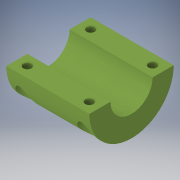
# Autodesk Inventor part: Slider Mount_B
Saved by Autodesk Inventor 2018 (Build 220112000, 112)
## iProperties
Created: 2018-01-05
Part Number: Slider Mount_B
Material: ABS Plastic
Document SubType Name: Modeling
Designer: njcfu
Density: 1.06 g/cm^3
Appearance: Olive Green
Author: njcfu
Autodesk Inventor part; units mm, degrees
sketch "Sketch2" plane through (0, 0, 0) normal (1, 0, 0) x (0, 1, 0)
  arc A0 (0, 12.7) -> (0, -12.7) centre (0, 0) ccw
  arc A1 (0, 25.4) -> (0, -25.4) centre (0, 0) ccw
  line L0 (0, -25.4) -> (0, -12.7)
  line L1 (0, 12.7) -> (0, 25.4)
  line L2 (0, 35.56) -> (0, -35.56) projected
  dimension "d5" = 180
  dimension "d122" = 180
  dimension "d123" = 12.7
  dimension "d124" = 25.4
  dimension "d125" = 12.7
  dimension "d127" = 0
  constraints: 4 end point, 4 point on circle, 2 centre point, 2 coincident
  measures "d122" angle of L2 L1
  measures "d123" radius of A0
  measures "d124" radius of A1
  measures "d125" distance of L1.start L1.end
  measures "d127" horizontal distance of L0.end L0.start
extrude "Extrusion1" add sketch "Sketch2" along normal mid plane 49.9999 contours A0 L0 A1 L1
ref_plane "Work Plane1" through (0, 0, 12.7) normal (0, 0, 1) x (1, 0, 0)
ref_plane "Work Plane2" through (0, -12.7, 0) normal (0, 1, 0) x (-1, 0, 0)
sketch "Sketch15" plane through (-25, 0, 25.4) normal (0, 1, 0) x (1, 0, 0)
  circle A0 centre (6.35, 6.35) radius 2.413
  circle A1 centre (43.6499, 6.35) radius 2.413
  circle A2 centre (43.6499, 44.45) radius 2.413
  circle A3 centre (6.35, 44.45) radius 2.413
  line L0 (0, 0) -> (0, 12.7) projected
  line L1 (49.9999, 12.7) -> (49.9999, 0) projected
  line L2 (49.9999, 50.8) -> (49.9999, 38.1) projected
  line L3 (0, 38.1) -> (0, 50.8) projected
  line L4 (49.9999, 50.8) -> (0, 50.8) projected
  line L5 (49.9999, 0) -> (0, 0) projected
  point P0 (25, 25.4)
  dimension "d128" = 4.826
  dimension "d129" = 4.826
  dimension "d130" = 4.826
  dimension "d131" = 4.826
  dimension "d132" = 6.35
  dimension "d133" = 6.35
  dimension "d134" = 6.35
  dimension "d135" = 6.35
  dimension "d136" = 6.35
  dimension "d137" = 6.35
  dimension "d138" = 6.35
  dimension "d139" = 6.35
  constraints: 4 centre point
  measures "d128" diameter of A3
  measures "d129" diameter of A2
  measures "d130" diameter of A1
  measures "d131" diameter of A0
  measures "d132" distance from line of L0 A0.centre
  measures "d133" distance from line of L1 A1.centre
  measures "d134" distance from line of L2 A2.centre
  measures "d135" distance from line of L3 A3.centre
  measures "d136" distance from line of L4 A3.centre
  measures "d137" distance from line of L4 A2.centre
  measures "d138" distance from line of L5 A1.centre
  measures "d139" distance from line of L5 A0.centre
extrude "Extrusion13" cut sketch "Sketch15" against normal up to next from surface at 0
ref_plane "Work Plane3" through (0, -13.5831, 0) normal (0, 1, 0) x (-1, 0, 0)
sketch "Sketch16" plane through (0, -13.5831, 0) normal (0, 1, 0) x (-1, 0, 0)
  circle A0 centre (-18.65, 19.05) radius 5.08
  circle A1 centre (-18.65, -19.05) radius 5.08
  circle A2 centre (18.65, -19.05) radius 5.08
  circle A3 centre (18.65, 19.05) radius 5.08
  circle A4 centre (-18.65, 19.05) radius 2.413 projected
  circle A5 centre (-18.65, -19.05) radius 2.413 projected
  circle A6 centre (18.65, -19.05) radius 2.413 projected
  circle A7 centre (18.65, 19.05) radius 2.413 projected
  point P0 (0, 0)
  dimension "d143" = 10.16
  dimension "d144" = 10.16
  dimension "d145" = 10.16
  dimension "d146" = 10.16
  constraints: 4 centre point, 4 concentric
  measures "d143" diameter of A0
  measures "d144" diameter of A3
  measures "d145" diameter of A2
  measures "d146" diameter of A1
extrude "Extrusion14" cut sketch "Sketch16" along normal blind 10.16 and the other way blind 12.7
body "Solid1"
